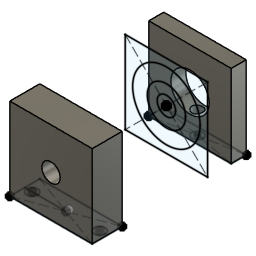
Thumb v35 (Autodesk Fusion 360 archive; units mm, degrees)
design "ThumbBrackets"
Autodesk Fusion 360 part; units mm, degrees
sketch "Sketch2" plane through (0, 0, 0) normal (0, 0, 1) x (1, 0, 0)
  circle A0 centre (0, 0) radius 2.45
  line L0 (11, 11) -> (-11, 11)
  line L1 (-11, 11) -> (-11, -11)
  line L2 (-11, -11) -> (11, -11)
  line L3 (11, -11) -> (11, 11)
  line L4 (11, 11) -> (-11, -11) construction
  line L5 (-11, 11) -> (11, -11) construction
  circle A1 centre (0, 0) radius 9
  circle A2 centre (0, 0) radius 5.1
  dimension "d17" = 4.9
  dimension "d18" = 22
  dimension "d90" = 18
  dimension "d104" = 10.2
  dimension "d121" = 22
  constraint coincident A0.centre A1.centre
  constraint horizontal L0
  constraint perpendicular L0 L1
  constraint parallel L0 L2
  constraint parallel L1 L3
  constraint coincident L4 A0.centre
  constraint coincident L5 A0.centre
  constraint concentric A0 A1
  measures "d17" diameter of A0
  measures "d18" distance of L1.end L2.end
  measures "d90" diameter of A1
  measures "d104" diameter of A2
  measures "d121" distance of L0.start L2.end
extrude "Extrude3" add sketch "Sketch2" against normal blind 4 from surface at -6.3 contours A0 | L0 L1 L2 L3 | A1 | A2 makes body 1
extrude "Extrude4" add sketch "Sketch2" along normal blind 4 from surface at 22.8 separate body contours L0 L1 L2 L3 makes body 2
extrude "Extrude5" add sketch "Sketch2" along normal blind 4 from surface at 26.8 contours L0 L1 L2 L3 | A1 | A2 bodies 2
sketch "Sketch7" plane through (0, -11, 0) normal (0, -1, 0) x (1, 0, 0)
  line L0 (-11, 22.8) -> (11, 22.8)
  line L1 (11, 22.8) -> (11, 30.8)
  line L2 (11, 30.8) -> (-11, 30.8)
  line L3 (-11, 30.8) -> (-11, 22.8)
  line L4 (11, 22.8) -> (-11, 22.8)
  line L5 (-11, 22.8) -> (-11, 30.8)
  line L6 (-11, 30.8) -> (11, 30.8)
  line L7 (11, 30.8) -> (11, 22.8)
  line L8 (11, 30.8) -> (-11, 22.8) construction
  line L9 (-11, 30.8) -> (11, 22.8) construction
  line L10 (0, 26.8) -> (-11, 26.8)
  circle A0 centre (-9, 26.8) radius 1.425
  line L11 (0, 26.8) -> (0, 26)
  circle A1 centre (9, 26.8) radius 1.425
  point P0 (0, 26.8)
  dimension "d98" = 2.85
  dimension "d99" = 9
  constraint horizontal L4
  constraint vertical L5
  constraint horizontal L6
  constraint vertical L7
  constraint coincident L2.end L3.start
  constraint coincident L0.end L1.start
  constraint midpoint L8 P0
  constraint midpoint L5 L10.end
  constraint coincident L10 A0.centre
  constraint coincident P0 L10.start
  constraint perpendicular L10 L11
  constraint symmetric A0 L11 A1
  measures "d98" diameter of A0
  measures "d99" distance of A0.centre P0
sketch "Sketch8" plane through (0, -11, 0) normal (0, -1, 0) x (1, 0, 0)
  line L0 (11, -6.3) -> (-11, -6.3)
  line L1 (-11, -6.3) -> (-11, -10.3)
  line L2 (-11, -10.3) -> (11, -10.3)
  line L3 (11, -10.3) -> (11, -6.3)
  line L4 (11, -10.3) -> (-11, -10.3)
  line L5 (-11, -10.3) -> (-11, -6.3)
  line L6 (-11, -6.3) -> (11, -6.3)
  line L7 (11, -6.3) -> (11, -10.3)
  line L8 (11, -10.3) -> (-11, -6.3) construction
  line L9 (11, -6.3) -> (-11, -10.3) construction
  circle A0 centre (0, -8.3) radius 1.425
  dimension "d72" = 2.85
  constraint horizontal L4
  constraint vertical L5
  constraint horizontal L6
  constraint vertical L7
  constraint coincident L0.end L1.start
  constraint coincident L2.end L3.start
  constraint midpoint L9 A0.centre
  measures "d72" diameter of A0
extrude "Extrude9" cut sketch "Sketch7" sketch "Sketch8" against normal blind 7 contours L10 A0 | L10 A0 | A1 of sketch 2 contours A0 bodies 1 2
extrude "Extrude11" cut sketch "Sketch2" against normal blind 10.5 contours A0 | A2 bodies 1
equation "d19 = -6 mm - 0.3 mm"
equation "d22 = 22.5 mm + 0.3 mm"
equation "d26 = 22.5 mm + 0.3 mm + 4 mm"
equation "d109 = -2 mm + 0.05 mm"

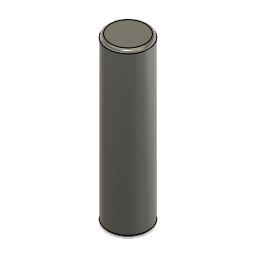
design "Finger Pin"
Autodesk Fusion 360 part; units mm, degrees
sketch "Sketch1" plane through (0, 0, 0) normal (0, 1, 0) x (1, 0, 0)
  circle A0 centre (0, 0) radius 2
  dimension "d1" = 4
  constraint coincident A0.centre origin
  measures "d1" diameter of A0
extrude "Extrude1" add sketch "Sketch1" along normal blind 16
fillet "Fillet1" radius 0.3 2 edges at (-1.8647, 16, 0.7232) (-1.8647, 0, 0.7232)

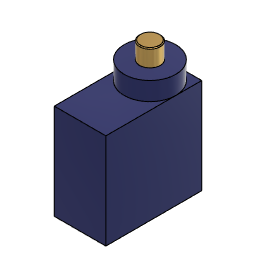
design "25105 Servo Clipped"
Autodesk Fusion 360 part; units mm, degrees
sketch "Sketch1" plane through (0, 0, 0) normal (0, 1, 0) x (1, 0, 0)
  line L0 (6.05, -16.15) -> (-6.05, -16.15)
  line L1 (-6.05, -16.15) -> (-6.05, 16.15)
  line L2 (-6.05, 16.15) -> (6.05, 16.15)
  line L3 (6.05, 16.15) -> (6.05, -16.15)
  line L4 (6.05, -16.15) -> (-6.05, 16.15) construction
  line L5 (-6.05, -16.15) -> (6.05, 16.15) construction
  line L6 (6.05, -11.25) -> (-6.05, -11.25)
  line L7 (-6.05, -11.25) -> (-6.05, 11.25)
  line L8 (-6.05, 11.25) -> (6.05, 11.25)
  line L9 (6.05, 11.25) -> (6.05, -11.25)
  line L10 (6.05, -11.25) -> (-6.05, 11.25) construction
  line L11 (-6.05, -11.25) -> (6.05, 11.25) construction
  line L12 (6.05, -13.85) -> (-6.05, -13.85) construction
  line L13 (-6.05, -13.85) -> (-6.05, 13.85) construction
  line L14 (-6.05, 13.85) -> (6.05, 13.85) construction
  line L15 (6.05, 13.85) -> (6.05, -13.85) construction
  line L16 (6.05, -13.85) -> (-6.05, 13.85) construction
  line L17 (-6.05, -13.85) -> (6.05, 13.85) construction
  line L18 (0, 16.15) -> (0, -16.15) construction
  circle A0 centre (0, 13.85) radius 1.1
  circle A1 centre (0, -13.85) radius 1.1
  line L19 (0, 13.85) -> (0, 5.15)
  circle A2 centre (0, 5.15) radius 2.43
  circle A3 centre (0, 5.15) radius 6.05
  circle A4 centre (0, 5.15) radius 1
  circle A5 centre (0, -0.9) radius 2.43
  line L20 (0.8, -16.1843) -> (-0.8, -16.1843)
  line L21 (-0.8, -16.1843) -> (-0.8, -13.7157)
  line L22 (-0.8, -13.7157) -> (0.8, -13.7157)
  line L23 (0.8, -13.7157) -> (0.8, -16.1843)
  line L24 (0.8, -16.1843) -> (-0.8, -13.7157) construction
  line L25 (-0.8, -16.1843) -> (0.8, -13.7157) construction
  line L26 (0.8, 16.15) -> (-0.8, 16.15)
  line L27 (-0.8, 16.15) -> (-0.8, 13.75)
  line L28 (-0.8, 13.75) -> (0.8, 13.75)
  line L29 (0.8, 13.75) -> (0.8, 16.15)
  line L30 (0.8, 16.15) -> (-0.8, 13.75) construction
  line L31 (-0.8, 16.15) -> (0.8, 13.75) construction
  point P0 (0, -14.95)
  point P1 (0, 14.95)
  dimension "d3" = 12.1
  dimension "d4" = 32.3
  dimension "d5" = 12.1
  dimension "d6" = 22.5
  dimension "d7" = 27.7
  dimension "d8" = 2.2
  dimension "d9" = 2.2
  dimension "d10" = 8.7
  dimension "d11" = 4.86
  dimension "d12" = 2
  dimension "d23" = 4.86
  dimension "d24" = 1.6
  dimension "d25" = 1.6
  constraint horizontal L0
  constraint perpendicular L0 L1
  constraint parallel L0 L2
  constraint parallel L1 L3
  constraint coincident L4 origin
  constraint coincident L5 origin
  constraint horizontal L6
  constraint perpendicular L6 L7
  constraint parallel L6 L8
  constraint parallel L7 L9
  constraint coincident L10 origin
  constraint coincident L11 origin
  constraint horizontal L12
  constraint perpendicular L12 L13
  constraint parallel L12 L14
  constraint parallel L13 L15
  constraint coincident L16 origin
  constraint coincident L17 origin
  constraint midpoint L2 L18.start
  constraint midpoint L0 L18.end
  constraint midpoint L14 A0.centre
  constraint midpoint L12 A1.centre
  constraint coincident A0.centre L19.start
  constraint perpendicular L8 L19
  constraint coincident L19.end A2.centre
  constraint concentric A2 A3
  constraint tangent L9 A3
  constraint tangent L15 A3
  constraint concentric A3 A4
  constraint coincident A3 A5.centre
  constraint coincident L18 A5.centre
  constraint horizontal L20
  constraint perpendicular L20 L21
  constraint parallel L20 L22
  constraint parallel L21 L23
  constraint coincident L24 P0
  constraint coincident L25 P0
  constraint coincident A1 P0
  constraint coincident L18 P0
  constraint horizontal L26
  constraint perpendicular L26 L27
  constraint parallel L26 L28
  constraint parallel L27 L29
  constraint coincident L30 P1
  constraint coincident L31 P1
  constraint coincident A0 P1
  constraint coincident L18 P1
  measures "d3" distance of L1.end L2.end
  measures "d4" distance of L0.end L1.end
  measures "d5" distance of L7.end L8.end
  measures "d6" distance of L6.end L7.end
  measures "d7" distance of L12.end L13.end
  measures "d8" diameter of A0
  measures "d9" diameter of A1
  measures "d10" distance of A0.centre L19.end
  measures "d11" diameter of A2
  measures "d12" diameter of A4
  measures "d23" diameter of A5
  measures "d24" distance of L21.end L22.end
  measures "d25" distance of L27.end L28.end
extrude "Extrude1" add sketch "Sketch1" against normal blind 15.7 contours L1 L3 L6 L7 L9 A3 A5 | L3 L8 L9 L19 A3 | A3 A5 | L1 L7 L8 L19 A3 | A3 A5 | A3 A5 | A2 | A4
extrude "Extrude2" add sketch "Sketch1" along normal blind 2.5 contours L1 L3 L6 L7 L9 A3 A5 | L3 L8 L9 L19 A3 | A3 A5 | L1 L7 L8 L19 A3 | A3 A5 | A3 A5 | A2 | A4
extrude "Extrude3" add sketch "Sketch1" along normal blind 6.7 contours L1 L3 L6 L7 L9 A3 A5 | L3 L8 L9 L19 A3 | A3 A5 | L1 L7 L8 L19 A3 | A3 A5 | A3 A5 | A2 | A4
extrude "Extrude4" add sketch "Sketch1" along normal blind 11 contours A3 A5 | A3 A5 | A2 | A4 picked at (2.681, 1.8148) picked at (0.4447, -0.0905)
extrude "Extrude5" add sketch "Sketch1" along normal blind 15 contours A2 | A4
fillet "Fillet1" radius 0.2 1 edges at (-2.2656, 15, -4.2713)
equation "d15 = 18.2 mm - 15.7 mm"
equation "d17 = 22.4 mm - 15.7 mm"
equation "d19 = 26.7 mm - 15.7 mm"
equation "d21 = 30.7 mm - 15.7 mm"
